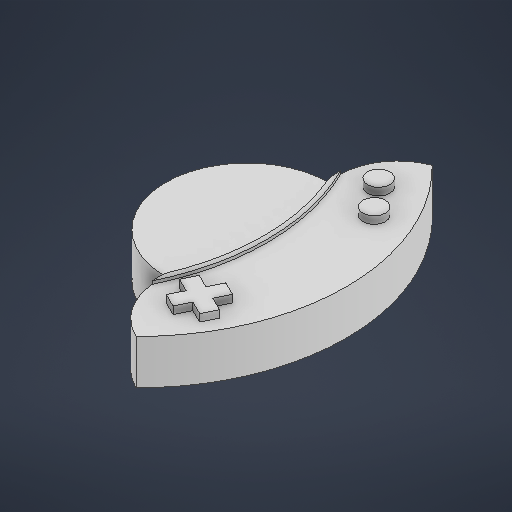
# Autodesk Inventor part: Alien tomadagi base design
Saved by Autodesk Inventor 2026.1 (Build 301233000, 233)
## iProperties
Created: 2026-01-10
Part Number: Alien tomadagi base design
Material: Generic
Document SubType Name: Modeling
Designer: WDsan
Density: 1 g/cm^3
Appearance: Default
Author: WDsan
Autodesk Inventor part; units mm, degrees
ref_plane "YZ Plane" through (0, 0, 0) normal (1, 0, 0) x (0, 1, 0)
ref_plane "XZ Plane" through (0, 0, 0) normal (0, 1, 0) x (-1, 0, 0)
ref_plane "XY Plane" through (0, 0, 0) normal (0, 0, 1) x (1, 0, 0)
sketch "Sketch3" plane through (0, 0, 0) normal (0, 1, 0) x (-1, 0, 0)
  arc A0 (0, 0) -> (0.0041, -20) centre (9.8, -9.998) ccw
  arc A1 (0.1922, -14.9904) -> (0.2252, -4.9905) centre (2.5, -9.998) ccw
  arc A2 (2.4909, -4.498) -> (0, 0) centre (-1.9245, -4.0045) ccw
  line L0 (9.8, -9.998) -> (2.5, -9.998)
  arc A3 (0.0041, -20) -> (2.5, -15.498) centre (-1.3582, -16.3019) ccw
  dimension "d4" = 20
  dimension "d7" = 10
  dimension "d10" = 7.3
  dimension "d11" = 0
  dimension "d12" = 2.5
  dimension "d13" = 5.5
  constraints: 10 point on circle, 4 centre point, 2 end point, 1 other
  measures "d4" distance of A0.start A0.end
  measures "d7" distance of A1.end A1.start
  measures "d10" distance of L0.start L0.end
  measures "d11" vertical distance of L0.end L0.start
  measures "d12" horizontal distance of A0.start L0.end
  measures "d13" radius of A1
extrude "Extrusion1" add sketch "Sketch3" along normal blind 3
sketch "Sketch4" plane through (0, 3, 0) normal (0, 1, 0) x (1, 0, 0)
  arc A0 (-2.4909, 4.498) -> (0, 0) centre (1.9245, 4.0045) ccw projected
  arc A1 (-0.0041, 20) -> (-2.5, 15.498) centre (1.3582, 16.3019) ccw projected
  line L0 (0, 0) -> (-0.0041, 20) construction
  circle A2 centre (-0.5544, 16.9415) radius 0.7578
  circle A3 centre (0.9535, 15.1232) radius 0.7578
  line L1 (-1.3792, 4.3024) -> (-0.9394, 5.2005)
  line L2 (-1.3792, 4.3024) -> (-0.4332, 4.6265) construction
  line L3 (-0.9394, 5.2005) -> (-0.0413, 4.7608)
  line L4 (-0.0413, 4.7608) -> (0.3984, 5.6589)
  line L5 (0.3984, 5.6589) -> (1.2965, 5.2191)
  line L6 (1.2965, 5.2191) -> (0.8568, 4.321)
  line L7 (0.8568, 4.321) -> (1.7549, 3.8812)
  line L8 (1.7549, 3.8812) -> (1.3151, 2.9831)
  line L9 (1.3151, 2.9831) -> (0.417, 3.4229)
  line L10 (0.417, 3.4229) -> (-0.0228, 2.5248)
  line L11 (-0.0228, 2.5248) -> (-0.9209, 2.9646)
  line L12 (-0.9209, 2.9646) -> (-0.4811, 3.8627)
  line L13 (-0.4811, 3.8627) -> (-1.3792, 4.3024)
  dimension "d20" = 1
  dimension "d21" = 45
  dimension "d22" = 1
  dimension "d24" = 1
  dimension "d25" = 1
  dimension "d26" = 1
  dimension "d27" = 1
  dimension "d28" = 1
  dimension "d29" = 1
  dimension "d30" = 1
  dimension "d32" = 1
  dimension "d33" = 1
  constraints: 28 end point, 6 perpendicular, 2 centre point, 2 point on line, 1 equal length
  measures "d20" distance of L1.start L1.end
  measures "d21" angle of L2 L1
  measures "d22" distance of L1.end L3.end
  measures "d24" distance of L3.end L4.end
  measures "d25" distance of L4.end L5.end
  measures "d26" distance of L5.end L6.end
  measures "d27" distance of L6.end L7.end
  measures "d28" distance of L7.end L8.end
  measures "d29" distance of L8.end L9.end
  measures "d30" distance of L9.end L10.end
  measures "d32" distance of L10.end L11.end
  measures "d33" distance of L11.end L12.end
extrude "Extrusion2" add sketch "Sketch4" along normal blind 0.5
sketch "Sketch5" plane through (0, 3, 0) normal (0, 1, 0) x (1, 0, 0)
  arc A0 (-2.5, 15.498) -> (-2.4909, 4.498) centre (-2.5, 9.998) ccw projected
  arc A1 (-2.4909, 4.498) -> (0, 0) centre (1.9245, 4.0045) ccw projected
  arc A2 (-0.0041, 20) -> (-2.5, 15.498) centre (1.3582, 16.3019) ccw projected
  arc A3 (-2.4909, 4.498) -> (-2.5, 15.498) centre (-15.3699, 9.9874) ccw
  arc A4 (-2.4988, 3.5873) -> (-2.5818, 16.3912) centre (-15.5502, 9.9049) ccw
  point P0 (-1.3699, 9.9989)
  point P1 (-1.0505, 9.9989)
  dimension "d37" = 14
  dimension "d38" = 14.5
  dimension "d39" = 0
  dimension "d40" = 0.3194
  constraints: 8 point on circle, 2 centre point
  measures "d37" radius of A3
  measures "d38" radius of A4
  measures "d39" vertical distance of point (-1.37, 9.999) point (-1.05, 9.999)
  measures "d40" distance of point (-1.37, 9.999) point (-1.05, 9.999)
extrude "Extrusion3" add sketch "Sketch5" along normal blind 0.2 contours A2 A4 A1 A3
body "Solid1"
